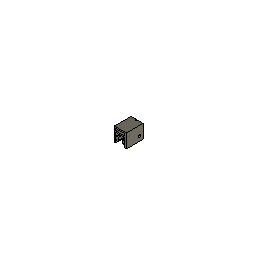
Frame_Support (Autodesk Fusion 360 design; units mm, degrees)
Autodesk Fusion 360 part; units mm, degrees
ref_plane "Plan de construction1" through (0, 3, 0) normal (0, 1, 0) x (0, 0, 1)
sketch "Esquisse1" plane through (0, 3, 0) normal (0, 1, 0) x (1, 0, 0)
  line L0 (-10, -4) -> (10, -4)
  line L1 (10, -4) -> (10, 0)
  line L2 (10, 0) -> (-10, 0)
  line L3 (-10, 0) -> (-10, -4)
  line L4 (-10.3, -4.3) -> (10.3, -4.3)
  line L5 (10.3, -4.3) -> (10.3, 0.3)
  line L6 (10.3, 0.3) -> (-10.3, 0.3)
  line L7 (-10.3, 0.3) -> (-10.3, -4.3)
  line L8 (-13.3, -7.3) -> (13.3, -7.3)
  line L9 (13.3, -7.3) -> (13.3, 23.3)
  line L10 (-13.3, 23.3) -> (-13.3, -7.3)
  line L11 (10, 3.3) -> (-10, 3.3)
  line L12 (-10, 23.3) -> (-10, 3.3)
  line L13 (10, 3.3) -> (10, 23.3)
  line L14 (13.3, 23.3) -> (10, 23.3)
  line L15 (-10, 23.3) -> (-13.3, 23.3)
  line L16 (-15, 13.3) -> (16, 13.3) construction
  line L17 (-5.9999, 8.8) -> (-7.4999, 8.8)
  line L18 (-7.4999, 8.8) -> (-7.4999, 10.5)
  line L19 (-7.4999, 10.5) -> (-9.9999, 10.5)
  line L20 (-9.9999, 10.5) -> (-9.9999, 16.1)
  line L21 (-9.9999, 16.1) -> (-7.4999, 16.1)
  line L22 (-7.4999, 16.1) -> (-7.4999, 17.8)
  line L23 (-7.4999, 17.8) -> (-5.9999, 17.8)
  line L24 (-5.9999, 17.8) -> (-4.5028, 16.0546)
  line L25 (-4.5028, 16.0546) -> (-4.5028, 10.4546)
  line L26 (-4.5028, 10.4546) -> (-5.9999, 8.8)
  line L27 (5.9999, 8.8) -> (7.4999, 8.8)
  line L28 (7.4999, 8.8) -> (7.4999, 10.5)
  line L29 (7.4999, 10.5) -> (9.9999, 10.5)
  line L30 (9.9999, 10.5) -> (9.9999, 16.1)
  line L31 (9.9999, 16.1) -> (7.4999, 16.1)
  line L32 (7.4999, 16.1) -> (7.4999, 17.8)
  line L33 (7.4999, 17.8) -> (5.9999, 17.8)
  line L34 (5.9999, 17.8) -> (4.5028, 16.0546)
  line L35 (4.5028, 10.4546) -> (5.9999, 8.8)
  line L36 (4.5028, 16.0546) -> (4.5028, 10.4546)
  line L37 (0, 205.75) -> (0, -209.25)
  dimension "d163" = 20
  dimension "d164" = 4
  dimension "d165" = 0.3
  dimension "d166" = 3
  dimension "d167" = 3
  dimension "d168" = 3
  dimension "d169" = 20
  dimension "d170" = 20
  dimension "d171" = 3.3
  dimension "d17" = 2.5
  dimension "d18" = 2.5
  dimension "d19" = 1.5
  dimension "d20" = 1.5
  dimension "d21" = 5.6
  dimension "d22" = 9
  dimension "d23" = 5.6
  dimension "d26" = 1.7
  constraint horizontal L0
  constraint vertical L1
  constraint horizontal L2
  constraint vertical L3
  constraint horizontal L8
  constraint vertical L9
  constraint horizontal L14
  constraint vertical L10
  constraint perpendicular L10 L11
  constraint coincident L12.start L14
  constraint perpendicular L12 L14
  constraint perpendicular L13 L14
  constraint collinear L14 L15
  constraint coincident origin L2
  constraint perpendicular L10 L16
  constraint horizontal L21
  constraint perpendicular L21 L22
  constraint perpendicular L22 L23
  constraint perpendicular L23 L25
  constraint perpendicular L17 L25
  constraint perpendicular L17 L18
  constraint perpendicular L19 L25
  constraint perpendicular L20 L21
  constraint symmetric L16 L19 L21
  measures "d163" distance of L0.start L0.end
  measures "d164" distance of L0.start L2.end
  measures "d166" distance of L5 L9
  measures "d167" distance of L4 L8
  measures "d168" distance of L6 L11
  measures "d169" distance of L11 L14
  measures "d170" distance of L12 L13
  measures "d171" distance of L9 L13
  measures "d17" distance of L20.end L21.end
  measures "d18" distance of L19.end L18.end
  measures "d19" distance of L17.start L17.end
  measures "d20" distance of L23.end L22.end
  measures "d21" distance of L19 L21
  measures "d22" distance of L17 L23
  measures "d23" distance of L25.end L24.end
  measures "d26" distance of L18.end L17.end
extrude "Extrusion1" add sketch "Esquisse1" along normal blind 37 contours L4 L6 L7 L8 L10 L11 L12 L15 L20 L37 | L4 L5 L6 L8 L9 L11 L13 L14 L30 L37 makes body 1
extrude "Extrusion2" add sketch "Esquisse1" along normal blind 20 separate body contours L13 L27 L28 L29 L30 L31 L32 L33 L34 L35 L36 | L12 L17 L18 L19 L20 L21 L22 L23 L24 L25 L26 makes body 2 at (-4.5028, 9.6667, -14.188) makes body 3 at (4.5028, 9.6667, -14.188)
sketch "Esquisse2" plane through (13.3, 0, 0) normal (1, 0, 0) x (0, 1, 0)
  line L0 (3, 7.3) -> (3, -23.3)
  line L1 (3, -23.3) -> (40, -23.3)
  line L2 (40, -23.3) -> (40, 7.3)
  line L3 (40, 7.3) -> (3, 7.3)
  line L4 (45, -13.3) -> (20, -13.3) construction
  line L5 (32.5, -5) -> (32.5, -27.6162) construction
  circle A0 centre (32.5, -13.3) radius 2.5
  dimension "d184" = 10
  dimension "d185" = 7.5
  dimension "d186" = 5
  constraint perpendicular L2 L4
  constraint perpendicular L1 L5
  constraint midpoint L4 A0.centre
  measures "d184" distance of L1 L4
  measures "d185" distance of L2 L5
  measures "d186" diameter of A0
extrude "Extrusion3" cut sketch "Esquisse2" against normal up to surface (26.6 mm away) contours A0 bodies 1
sketch "Esquisse3" plane through (0, 0, 7.3) normal (0, 0, 1) x (-1, 0, 0)
  line L0 (13.3, -3) -> (-13.3, -3)
  line L1 (-13.3, -3) -> (-13.3, -40)
  line L2 (-13.3, -40) -> (13.3, -40)
  line L3 (13.3, -40) -> (13.3, -3)
  line L4 (20, -38.5) -> (-20, -38.5) construction
  line L5 (2.5, -39) -> (-2.5, -39)
  line L6 (-2.5, -39) -> (-2.5, -38)
  line L7 (-2.5, -38) -> (2.5, -38)
  line L8 (2.5, -38) -> (2.5, -39)
  line L9 (0, -42) -> (0, -32) construction
  line L10 (-13.3, -40) -> (-13.3, -3)
  dimension "d190" = 5
  dimension "d191" = 1
  dimension "d192" = 1
  constraint perpendicular L3 L4
  constraint horizontal L5
  constraint vertical L6
  constraint horizontal L7
  constraint vertical L8
  constraint symmetric L4 L5 L7
  constraint vertical L9
  constraint symmetric L6 L8 L9
  measures "d190" distance of L5.start L5.end
  measures "d191" distance of L5.start L7.end
  measures "d192" distance of L2 L5
extrude "Extrusion4" add sketch "Esquisse3" along normal blind 0.5 contours L5 L6 L7 L8 bodies 1
fillet "Congé1" radius 0.5 2 edges at (0, 38, 7.8) (0, 39, 7.8) on bodies 1
